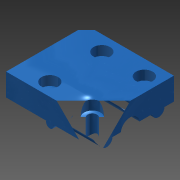
# Autodesk Inventor part: YAxisMotorCap
Saved by Autodesk Inventor 2015 (Build 190159000, 159)
## iProperties
Created: 2014-08-09
Part Number: YAxisMotorCap
Material: ABS Plastic
Document SubType Name: Modeling
Designer: Jack
Density: 1.06 g/cm^3
Appearance: Cyan
Author: Jack
Autodesk Inventor part; units mm, degrees
ref_plane "YZ Plane" through (0, 0, 0) normal (1, 0, 0) x (0, 1, 0)
ref_plane "XZ Plane" through (0, 0, 0) normal (0, 1, 0) x (-1, 0, 0)
ref_plane "XY Plane" through (0, 0, 0) normal (0, 0, 1) x (1, 0, 0)
sketch "Sketch1" plane through (0, 0, 0) normal (0, 0, 1) x (1, 0, 0)
  line L0 (0, 0) -> (37, 0)
  line L1 (37, 0) -> (37, 34)
  line L2 (37, 34) -> (0, 34)
  line L3 (0, 34) -> (0, 0)
  dimension "d0" = 37
  dimension "d1" = 34
  constraints: 8 end point, 2 parallel, 1 horizontal, 1 perpendicular
  measures "d0" distance of L1.end L2.end
  measures "d1" distance of L0.end L1.end
extrude "Extrusion1" add sketch "Sketch1" along normal blind 9.5
sketch "Sketch2" plane through (37, 0, 0) normal (1, 0, 0) x (0, 0, -1)
  line L0 (0, 0) -> (0, 34) projected
  line L1 (0, 0) -> (-9.5, 0) projected
  circle A0 centre (0.5, 15.5) radius 4
  dimension "d4" = 8
  dimension "d5" = 15.5
  dimension "d6" = 0.5
  constraints: 1 centre point
  measures "d4" diameter of A0
  measures "d5" distance from line of L1 A0.centre
  measures "d6" distance from line of L0 A0.centre
extrude "Extrusion2" cut sketch "Sketch2" against normal up to surface (37 mm away)
sketch "Sketch4" plane through (37, 0, 9.5) normal (1, 0, 0) x (0, 0, -1)
  line L0 (9.5, 19.4686) -> (9.5, 34) projected
  line L1 (9.5, 0) -> (0, 0) projected
  line L2 (9.5, 0) -> (9.5, 11.5314) projected
  circle A0 centre (9.5, 27.5) radius 2.5
  circle A1 centre (9.5, 5.5) radius 2.5
  dimension "d19" = 5
  dimension "d20" = 5
  dimension "d21" = 5.5
  dimension "d45" = 27.5
  constraints: 2 centre point, 2 point on line
  measures "d19" diameter of A0
  measures "d20" diameter of A1
  measures "d21" distance from line of L1 A1.centre
  measures "d45" distance from line of L1 A0.centre
extrude "Extrusion4" add sketch "Sketch4" against normal blind 30
sketch "Sketch3" plane through (0, 0, 9.5) normal (0, 0, 1) x (1, 0, 0)
  line L0 (0, 0) -> (37, 0) projected
  line L1 (37, 0) -> (37, 34) projected
  circle A0 centre (31, 5.5) radius 2
  circle A1 centre (31, 27.5) radius 2
  circle A2 centre (13, 5.5) radius 2
  circle A3 centre (13, 27.5) radius 2
  dimension "d9" = 4
  dimension "d10" = 6
  dimension "d11" = 5.5
  dimension "d12" = 27.5
  dimension "d13" = 4
  dimension "d15" = 24
  dimension "d16" = 4
  constraints: 4 centre point, 2 horizontal alignment, 2 vertical alignment, 1 equal radius
  measures "d9" diameter of A0
  measures "d10" distance from line of L1 A0.centre
  measures "d11" distance from line of L0 A0.centre
  measures "d12" distance from line of L0 A1.centre
  measures "d13" diameter of A2
  measures "d15" distance from line of L1 A2.centre
  measures "d16" diameter of A3
extrude "Extrusion3" cut sketch "Sketch3" against normal up to next
sketch "Sketch5" plane through (0, 0, 9.5) normal (-1, 0, 0) x (0, 0, 1)
  line L0 (-9.5, 11.5314) -> (-9.5, 0) projected
  line L1 (-9.5, 0) -> (0, 0) projected
  circle A0 centre (-10, 27.5) radius 4.25
  circle A1 centre (-10, 5.5) radius 4.25
  dimension "d25" = 8.5
  dimension "d26" = 8.5
  dimension "d27" = 0.5
  dimension "d28" = 5.5
  dimension "d46" = 27.5
  constraints: 2 centre point, 1 vertical alignment
  measures "d25" diameter of A0
  measures "d26" diameter of A1
  measures "d27" distance from line of L0 A1.centre
  measures "d28" distance from line of L1 A1.centre
  measures "d46" distance from line of L1 A0.centre
extrude "Extrusion5" cut sketch "Sketch5" against normal blind 7
sketch "Sketch6" plane through (0, 34, 0) normal (0, 1, 0) x (1, 0, 0)
  line L0 (37, 0) -> (0, 0) projected
  line L1 (37, 0) -> (37, -9.5) projected
  circle A0 centre (18.5, 0.5) radius 5.5
  dimension "d32" = 11
  dimension "d33" = 0.5
  dimension "d34" = 18.5
  constraints: 1 centre point
  measures "d32" diameter of A0
  measures "d33" distance from line of L0 A0.centre
  measures "d34" distance from line of L1 A0.centre
extrude "Extrusion6" cut sketch "Sketch6" against normal blind 1
sketch "Sketch7" plane through (0, 0, 0) normal (0, -1, 0) x (1, 0, 0)
  line L0 (0, 0) -> (37, 0) projected
  line L1 (37, 0) -> (37, 9.5) projected
  circle A0 centre (18.5, -0.5) radius 1.6
  dimension "d37" = 3.2
  dimension "d38" = 0.5
  dimension "d39" = 18.5
  constraints: 1 centre point
  measures "d37" diameter of A0
  measures "d38" distance from line of L0 A0.centre
  measures "d39" distance from line of L1 A0.centre
extrude "Extrusion7" add sketch "Sketch7" against normal blind 6
sketch "Sketch8" plane through (0, 0, 9.5) normal (0, 0, 1) x (1, 0, 0)
  circle A0 centre (13, 5.5) radius 2 projected
  circle A1 centre (31, 5.5) radius 2 projected
  circle A2 centre (31, 27.5) radius 2 projected
  circle A3 centre (13, 27.5) radius 2 projected
  circle A4 centre (13, 27.5) radius 3.5
  circle A5 centre (31, 27.5) radius 3.5
  circle A6 centre (31, 5.5) radius 3.5
  circle A7 centre (13, 5.5) radius 3.5
  dimension "d42" = 7
  constraints: 4 centre point, 4 coincident, 3 equal radius
  measures "d42" diameter of A4
extrude "Extrusion8" cut sketch "Sketch8" against normal blind 4
body "Solid1"
